Autodesk Fusion 360 part; units mm, degrees
(part 2 of 2)
sketch "Skizze1" plane through (0, 0, 0) normal (0, 0, 1) x (1, 0, 0)
  line L0 (-200, 300) -> (200, 300)
  line L1 (200, 300) -> (200, -300)
  line L2 (200, -300) -> (-200, -300)
  line L3 (-200, -300) -> (-200, 300)
  line L4 (-200, 300) -> (200, -300) construction
  line L5 (200, 300) -> (-200, -300) construction
  dimension "d1" = 600
  dimension "d2" = 400
  constraint horizontal L0
  constraint perpendicular L0 L1
  constraint parallel L0 L2
  constraint parallel L1 L3
  constraint coincident L4 origin
  constraint coincident L5 origin
  measures "d1" distance of L0.end L1.end
  measures "d2" distance of L0.start L0.end
extrude "Extrusion1" add sketch "Skizze1" along normal blind 200
fillet "Abrundung1" radius 40 4 edges at (200, -300, 100) (-200, -300, 100) (200, 300, 100) (-200, 300, 100)
fillet "Abrundung2" radius 5 2 faces at (-66.6667, -86.6667, 200) (-66.6667, -86.6667, 0)
sketch "Skizze2" plane through (0, 0, 200) normal (0, 0, 1) x (-1, 0, 0)
  arc A0 (160, -295) -> (195, -260) centre (160, -260) ccw
  line L0 (195, -260) -> (195, 260)
  arc A1 (195, 260) -> (160, 295) centre (160, 260) ccw
  line L1 (160, 295) -> (-160, 295)
  arc A2 (-160, 295) -> (-195, 260) centre (-160, 260) ccw
  line L2 (-195, 260) -> (-195, -260)
  arc A3 (-195, -260) -> (-160, -295) centre (-160, -260) ccw
  line L3 (-160, -295) -> (160, -295)
  line L4 (-125, -200) -> (125, -200)
  line L5 (125, -200) -> (125, 200)
  line L6 (125, 200) -> (-125, 200)
  line L7 (-125, 200) -> (-125, -200)
  line L8 (-125, -200) -> (125, 200) construction
  line L9 (125, -200) -> (-125, 200) construction
  dimension "d9" = 250
  dimension "d10" = 400
  constraint horizontal L4
  constraint perpendicular L4 L5
  constraint parallel L4 L6
  constraint parallel L5 L7
  constraint coincident L8 origin
  constraint coincident L9 origin
  measures "d9" distance of L4.start L4.end
  measures "d10" distance of L4.start L6.end
hole "Bohrung1" at (125, 200, 200) at (125, -200, 200) direction (0, 0, -1) diameter 30 depth 5 tip angle 180

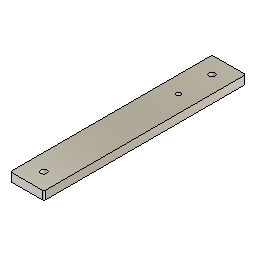
design "StrebeLängs1Cell"
Autodesk Fusion 360 part; units mm, degrees
sketch "Skizze1" plane through (0, 0, 0) normal (0, 0, 1) x (1, 0, 0)
  line L0 (-20, 120) -> (20, 120)
  line L1 (20, 120) -> (20, -120)
  line L2 (20, -120) -> (-20, -120)
  line L3 (-20, -120) -> (-20, 120)
  line L4 (-20, 120) -> (20, -120) construction
  line L5 (20, 120) -> (-20, -120) construction
  dimension "d1" = 40
  dimension "d2" = 240
  constraint horizontal L0
  constraint perpendicular L0 L1
  constraint parallel L0 L2
  constraint parallel L1 L3
  constraint coincident L4 origin
  constraint coincident L5 origin
  measures "d1" distance of L1.end L2.end
  measures "d2" distance of L0.end L1.end
extrude "Extrusion1" add sketch "Skizze1" along normal blind 10
sketch "Skizze2" plane through (0, 0, 10) normal (0, 0, 1) x (-1, 0, 0)
  line L0 (20, 120) -> (-20, 120)
  line L1 (-20, 120) -> (-20, -120)
  line L2 (-20, -120) -> (20, -120)
  line L3 (20, -120) -> (20, 120)
  line L4 (0, -100) -> (0, 100)
  dimension "d5" = 20
  dimension "d6" = 20
  constraint perpendicular L0 L4
  constraint coincident origin L4
  measures "d5" distance of L0 L4.end
  measures "d6" distance of L2 L4.start
hole "Bohrung1" at (0, 100, 10) at (0, -100, 10) direction (0, 0, -1) diameter 7 depth 60 tip angle 118
fillet "Abrundung1" radius 2 4 edges at (-20, -120, 5) (20, -120, 5) (20, 120, 5) (-20, 120, 5)
sketch "Skizze3" plane through (0, 0, 10) normal (0, 0, 1) x (-1, 0, 0)
  circle A0 centre (0, -100) radius 3.5
  circle A1 centre (0, 100) radius 3.5
  arc A2 (18, -120) -> (20, -118) centre (18, -118) ccw
  line L0 (20, -118) -> (20, 118)
  arc A3 (20, 118) -> (18, 120) centre (18, 118) ccw
  line L1 (18, 120) -> (-18, 120)
  arc A4 (-18, 120) -> (-20, 118) centre (-18, 118) ccw
  line L2 (-20, 118) -> (-20, -118)
  arc A5 (-20, -118) -> (-18, -120) centre (-18, -118) ccw
  line L3 (-18, -120) -> (18, -120)
  circle A6 centre (0, -60) radius 9.1766
  dimension "d13" = 60
  measures "d13" distance of origin A6.centre
hole "Bohrung2" at (0, 60, 10) direction (0, 0, -1) diameter 5.035 depth 10 tip angle 118
thread "Gewinde1" "ISO Metric profile 6.0 M6x1 6H"

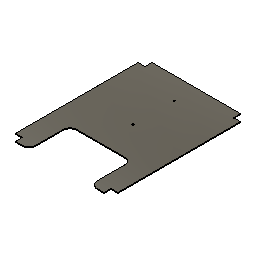
design "MittelPlatte"
Autodesk Fusion 360 part; units mm, degrees
sketch "Skizze1" plane through (0, 0, 0) normal (0, 0, 1) x (1, 0, 0)
  line L0 (-300, 400) -> (300, 400)
  line L1 (300, 400) -> (300, -400)
  line L2 (300, -400) -> (-300, -400)
  line L3 (-300, -400) -> (-300, 400)
  line L4 (-300, 400) -> (300, -400) construction
  line L5 (300, 400) -> (-300, -400) construction
  line L6 (-259.5, 359.5) -> (259.5, 359.5)
  line L7 (259.5, 359.5) -> (259.5, -359.5)
  line L8 (259.5, -359.5) -> (-259.5, -359.5)
  line L9 (-259.5, -359.5) -> (-259.5, 359.5)
  line L10 (-259.5, 359.5) -> (259.5, -359.5) construction
  line L11 (259.5, 359.5) -> (-259.5, -359.5) construction
  line L12 (-300, 400) -> (-259.5, 400)
  line L13 (-259.5, 400) -> (-259.5, 359.5)
  line L14 (-259.5, 359.5) -> (-300, 359.5)
  line L15 (-300, 359.5) -> (-300, 400)
  line L16 (259.5, 359.5) -> (300, 359.5)
  line L17 (300, 359.5) -> (300, 400)
  line L18 (300, 400) -> (259.5, 400)
  line L19 (259.5, 400) -> (259.5, 359.5)
  line L20 (-259.5, -359.5) -> (-300, -359.5)
  line L21 (-300, -359.5) -> (-300, -400)
  line L22 (-300, -400) -> (-259.5, -400)
  line L23 (-259.5, -400) -> (-259.5, -359.5)
  line L24 (259.5, -359.5) -> (300, -359.5)
  line L25 (300, -359.5) -> (300, -400)
  line L26 (300, -400) -> (259.5, -400)
  line L27 (259.5, -400) -> (259.5, -359.5)
  dimension "d1" = 600
  dimension "d2" = 800
  dimension "d3" = 40.5
  dimension "d4" = 40.5
  constraint horizontal L0
  constraint perpendicular L0 L1
  constraint parallel L0 L2
  constraint parallel L1 L3
  constraint coincident L4 origin
  constraint coincident L5 origin
  constraint horizontal L6
  constraint perpendicular L6 L7
  constraint parallel L6 L8
  constraint parallel L7 L9
  constraint coincident L10 origin
  constraint coincident L11 origin
  constraint horizontal L12
  constraint vertical L13
  constraint horizontal L14
  constraint vertical L15
  constraint horizontal L16
  constraint vertical L17
  constraint horizontal L18
  constraint vertical L19
  constraint horizontal L20
  constraint vertical L21
  constraint horizontal L22
  constraint vertical L23
  constraint horizontal L24
  constraint vertical L25
  constraint horizontal L26
  constraint vertical L27
  constraint coincident L0.end L17
  constraint coincident L0 L1.start
  measures "d1" distance of L1.end L2.end
  measures "d2" distance of L0.end L1.end
  measures "d3" distance of L0 L6
  measures "d4" distance of L3 L9
extrude "Extrusion1" add sketch "Skizze1" along normal blind 5 contours L0 L6 L13 L19 | L3 L9 L14 L20 | L6 L7 L8 L9 | L1 L7 L16 L24 | L2 L8 L23 L27
sketch "Skizze4" plane through (0, 0, 5) normal (0, 0, 1) x (-1, 0, 0)
  line L0 (259.5, 400) -> (-259.5, 400)
  line L1 (-259.5, 400) -> (-259.5, 359.5)
  line L2 (-259.5, 359.5) -> (-300, 359.5)
  line L3 (-300, 359.5) -> (-300, -359.5)
  line L4 (-300, -359.5) -> (-259.5, -359.5)
  line L5 (-259.5, -359.5) -> (-259.5, -400)
  line L6 (-259.5, -400) -> (259.5, -400)
  line L7 (259.5, -400) -> (259.5, -359.5)
  line L8 (259.5, -359.5) -> (300, -359.5)
  line L9 (300, -359.5) -> (300, 359.5)
  line L10 (300, 359.5) -> (259.5, 359.5)
  line L11 (259.5, 359.5) -> (259.5, 400)
  line L12 (0, -270) -> (0, -30)
  dimension "d23" = 240
  dimension "d24" = 130
  constraint vertical L12
  constraint coincident origin L12
  measures "d23" distance of L12.start L12.end
  measures "d24" distance of L6 L12.start
hole "Bohrung3" at (0, 270, 5) at (0, 30, 5) direction (0, 0, -1) diameter 10 depth 10 tip angle 118
sketch "Skizze6" plane through (0, 0, 5) normal (0, 0, 1) x (-1, 0, 0)
  line L0 (259.5, -400) -> (259.5, -359.5)
  line L1 (259.5, -359.5) -> (300, -359.5)
  line L2 (300, -359.5) -> (300, 359.5)
  line L3 (300, 359.5) -> (259.5, 359.5)
  line L4 (259.5, 359.5) -> (259.5, 400)
  line L5 (259.5, 400) -> (-259.5, 400)
  line L6 (-259.5, 400) -> (-259.5, 359.5)
  line L7 (-259.5, 359.5) -> (-300, 359.5)
  line L8 (-300, 359.5) -> (-300, -359.5)
  line L9 (-300, -359.5) -> (-259.5, -359.5)
  line L10 (-259.5, -359.5) -> (-259.5, -400)
  line L11 (-259.5, -400) -> (259.5, -400)
  circle A0 centre (0, -270) radius 5
  circle A1 centre (0, -30) radius 5
  line L12 (180, 400) -> (-180, 400)
  line L13 (-180, 400) -> (-180, 160)
  line L14 (-180, 160) -> (180, 160)
  line L15 (180, 160) -> (180, 400)
  line L16 (259.75, 160.25) -> (300.25, 160.25)
  line L17 (300.25, 160.25) -> (300.25, 119.75)
  line L18 (300.25, 119.75) -> (259.75, 119.75)
  line L19 (259.75, 119.75) -> (259.75, 160.25)
  line L20 (259.75, 160.25) -> (300.25, 119.75) construction
  line L21 (300.25, 160.25) -> (259.75, 119.75) construction
  line L22 (-300.25, 160.25) -> (-259.75, 160.25)
  line L23 (-259.75, 160.25) -> (-259.75, 119.75)
  line L24 (-259.75, 119.75) -> (-300.25, 119.75)
  line L25 (-300.25, 119.75) -> (-300.25, 160.25)
  line L26 (-300.25, 160.25) -> (-259.75, 119.75) construction
  line L27 (-259.75, 160.25) -> (-300.25, 119.75) construction
  point P0 (280, 140)
  point P1 (-280, 140)
  dimension "d30" = 560
  dimension "d31" = 120
  dimension "d32" = 120
  dimension "d37" = 40.5
  dimension "d38" = 40.5
  dimension "d39" = 20
  dimension "d40" = 20
  dimension "d42" = 20
  dimension "d43" = 20
  constraint horizontal L12
  constraint vertical L13
  constraint horizontal L14
  constraint vertical L15
  constraint coincident L5 L12.start
  constraint horizontal L16
  constraint perpendicular L16 L17
  constraint parallel L16 L18
  constraint parallel L17 L19
  constraint coincident L20 P0
  constraint coincident L21 P0
  constraint horizontal L22
  constraint perpendicular L22 L23
  constraint parallel L22 L24
  constraint parallel L23 L25
  constraint coincident L26 P1
  constraint coincident L27 P1
  constraint equal L18 L24
  constraint equal L19 L23
  measures "d30" distance of L11 L14
  measures "d31" distance of L2 L15
  measures "d32" distance of L8 L13
  measures "d37" distance of L17.end L18.end
  measures "d38" distance of L16.end L17.end
  measures "d39" distance of L2 P0
  measures "d40" distance of L8 P1
  measures "d42" distance of L14 P1
  measures "d43" distance of L14 P0
extrude "Extrusion2" cut sketch "Skizze6" against normal blind 10 contours L2 L16 L17 L18 | L8 L22 L24 L25 | L5 L12 L13 L14 L15
fillet "Abrundung2" radius 40 4 edges at (-180, -160, 2.5) (180, -160, 2.5) (-180, -400, 2.5) (180, -400, 2.5)
fillet "Abrundung1" radius 2 12 edges at (-300, -359.5, 2.5) (-259.5, -359.5, 2.5) (-259.5, -400, 2.5) (259.5, -400, 2.5) (259.5, -359.5, 2.5) (300, -359.5, 2.5) (300, 359.5, 2.5) (259.5, 359.5, 2.5) (259.5, 400, 2.5) (-300, 359.5, 2.5) (-259.5, 359.5, 2.5) (-259.5, 400, 2.5)
sketch "Skizze5" plane through (0, 0, 5) normal (0, 0, 1) x (-1, 0, 0)
  arc A0 (257.5, -400) -> (259.5, -398) centre (257.5, -398) ccw
  line L0 (259.5, -398) -> (259.5, -361.5)
  arc A1 (261.5, -359.5) -> (259.5, -361.5) centre (261.5, -361.5) ccw
  line L1 (261.5, -359.5) -> (298, -359.5)
  arc A2 (298, -359.5) -> (300, -357.5) centre (298, -357.5) ccw
  line L2 (300, -357.5) -> (300, 357.5)
  arc A3 (300, 357.5) -> (298, 359.5) centre (298, 357.5) ccw
  line L3 (298, 359.5) -> (261.5, 359.5)
  arc A4 (259.5, 361.5) -> (261.5, 359.5) centre (261.5, 361.5) ccw
  line L4 (259.5, 361.5) -> (259.5, 398)
  arc A5 (259.5, 398) -> (257.5, 400) centre (257.5, 398) ccw
  line L5 (-222, 400) -> (-257.5, 400)
  arc A6 (-257.5, 400) -> (-259.5, 398) centre (-257.5, 398) ccw
  line L6 (-259.5, 398) -> (-259.5, 361.5)
  arc A7 (-261.5, 359.5) -> (-259.5, 361.5) centre (-261.5, 361.5) ccw
  line L7 (-261.5, 359.5) -> (-298, 359.5)
  arc A8 (-298, 359.5) -> (-300, 357.5) centre (-298, 357.5) ccw
  line L8 (-300, 357.5) -> (-300, -357.5)
  arc A9 (-300, -357.5) -> (-298, -359.5) centre (-298, -357.5) ccw
  line L9 (-298, -359.5) -> (-261.5, -359.5)
  arc A10 (-259.5, -361.5) -> (-261.5, -359.5) centre (-261.5, -361.5) ccw
  line L10 (-259.5, -361.5) -> (-259.5, -398)
  arc A11 (-259.5, -398) -> (-257.5, -400) centre (-257.5, -398) ccw
  line L11 (-257.5, -400) -> (257.5, -400)
  circle A12 centre (0, -270) radius 5
  circle A13 centre (0, -30) radius 5
  arc A14 (-220, 398) -> (-222, 400) centre (-222, 398) ccw
  line L12 (257.5, 400) -> (222, 400)
  arc A15 (222, 400) -> (220, 398) centre (222, 398) ccw
  line L13 (220, 398) -> (220, 240)
  arc A16 (180, 200) -> (220, 240) centre (180, 240) ccw
  line L14 (180, 200) -> (-180, 200)
  arc A17 (-220, 240) -> (-180, 200) centre (-180, 240) ccw
  line L15 (-220, 240) -> (-220, 398)

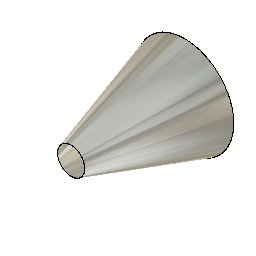
design "Trichter_groß"
Autodesk Fusion 360 part; units mm, degrees
sketch "Skizze1" plane through (0, 0, 0) normal (1, 0, 0) x (0, 1, 0)
  line L0 (-580, 70) -> (-580, 0)
  line L1 (-580, 0) -> (0, 0)
  line L2 (0, 250) -> (0, 0)
  line L3 (-580, 70) -> (0, 250)
  line L4 (-230, 0) -> (-230, 178.6207)
  dimension "d3" = 250
  dimension "d4" = 70
  dimension "d5" = 580
  dimension "d8" = 230
  constraint vertical L0
  constraint perpendicular L0 L1
  constraint perpendicular L1 L2
  constraint coincident L1.end L2
  constraint coincident L2.end L1
  constraint coincident L1 L4.start
  constraint coincident L3 L4.end
  constraint perpendicular L1 L4
  measures "d3" distance of L1.end L2.start
  measures "d4" vertical distance of L1.end L0.start
  measures "d5" distance of L1.end L0
  measures "d8" distance of L2 L4
revolve "Drehen1" add sketch "Skizze1" angle 360 about axis through (0, -580, 0) along (0, 1, 0)
shell "Schale1" thickness 1 removed faces 2 at (33.8089, -580, -13.7168) at (54.8247, 0, 36.3167)

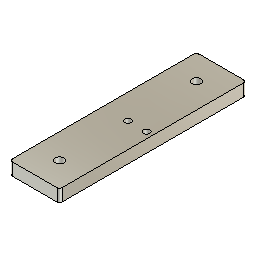
design "StrebeQuer1Cell"
Autodesk Fusion 360 part; units mm, degrees
sketch "Skizze1" plane through (0, 0, 0) normal (0, 0, 1) x (1, 0, 0)
  line L0 (-20, 75) -> (20, 75)
  line L1 (20, 75) -> (20, -75)
  line L2 (20, -75) -> (-20, -75)
  line L3 (-20, -75) -> (-20, 75)
  line L4 (-20, 75) -> (20, -75) construction
  line L5 (20, 75) -> (-20, -75) construction
  dimension "d1" = 40
  dimension "d2" = 150
  constraint horizontal L0
  constraint perpendicular L0 L1
  constraint parallel L0 L2
  constraint parallel L1 L3
  constraint coincident L4 origin
  constraint coincident L5 origin
  measures "d1" distance of L1.end L2.end
  measures "d2" distance of L0.end L1.end
extrude "Extrusion1" add sketch "Skizze1" along normal blind 10
sketch "Skizze2" plane through (0, 0, 10) normal (0, 0, 1) x (-1, 0, 0)
  line L0 (20, 75) -> (-20, 75)
  line L1 (-20, 75) -> (-20, -75)
  line L2 (-20, -75) -> (20, -75)
  line L3 (20, -75) -> (20, 75)
  line L4 (0, -55) -> (0, 55)
  dimension "d5" = 20
  dimension "d6" = 20
  constraint perpendicular L0 L4
  constraint coincident origin L4
  measures "d5" distance of L0 L4.end
  measures "d6" distance of L2 L4.start
hole "Bohrung1" at (0, 55, 10) at (0, -55, 10) direction (0, 0, -1) diameter 7 depth 60 tip angle 118
fillet "Abrundung1" radius 2 4 edges at (-20, -75, 5) (20, -75, 5) (20, 75, 5) (-20, 75, 5)
sketch "Skizze3" plane through (0, 0, 10) normal (0, 0, 1) x (-1, 0, 0)
  circle A0 centre (0, -55) radius 3.5
  circle A1 centre (0, 55) radius 3.5
  arc A2 (18, -75) -> (20, -73) centre (18, -73) ccw
  line L0 (20, -73) -> (20, 73)
  arc A3 (20, 73) -> (18, 75) centre (18, 73) ccw
  line L1 (18, 75) -> (-18, 75)
  arc A4 (-18, 75) -> (-20, 73) centre (-18, 73) ccw
  line L2 (-20, 73) -> (-20, -73)
  arc A5 (-20, -73) -> (-18, -75) centre (-18, -73) ccw
  line L3 (-18, -75) -> (18, -75)
  line L4 (-15, 0) -> (0, 0)
  dimension "d12" = 15
  dimension "d13" = 15
  constraint horizontal L4
  constraint coincident origin L4
  measures "d12" distance of L4.start L4.end
  measures "d13" distance of L4.end L4.start
hole "Bohrung2" at (15, 0, 10) at (0, 0, 10) direction (0, 0, -1) diameter 5 depth 10 tip angle 118

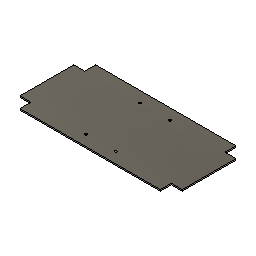
design "WaagePlatte"
Autodesk Fusion 360 part; units mm, degrees
sketch "Skizze1" plane through (0, 0, 0) normal (0, 0, 1) x (1, 0, 0)
  line L0 (-300, 140) -> (300, 140)
  line L1 (300, 140) -> (300, -140)
  line L2 (300, -140) -> (-300, -140)
  line L3 (-300, -140) -> (-300, 140)
  line L4 (-300, 140) -> (300, -140) construction
  line L5 (300, 140) -> (-300, -140) construction
  dimension "d1" = 600
  dimension "d2" = 280
  constraint horizontal L0
  constraint perpendicular L0 L1
  constraint parallel L0 L2
  constraint parallel L1 L3
  constraint coincident L4 origin
  constraint coincident L5 origin
  measures "d1" distance of L1.end L2.end
  measures "d2" distance of L0.end L1.end
extrude "Extrusion1" add sketch "Skizze1" along normal blind 5
sketch "Skizze2" plane through (0, 0, 5) normal (0, 0, 1) x (-1, 0, 0)
  line L0 (300, 140) -> (-300, 140)
  line L1 (-300, 140) -> (-300, -140)
  line L2 (-300, -140) -> (300, -140)
  line L3 (300, -140) -> (300, 140)
  line L4 (259.5, -99.5) -> (-259.5, -99.5)
  line L5 (-259.5, -99.5) -> (-259.5, 99.5)
  line L6 (-259.5, 99.5) -> (259.5, 99.5)
  line L7 (259.5, 99.5) -> (259.5, -99.5)
  line L8 (259.5, -99.5) -> (-259.5, 99.5) construction
  line L9 (-259.5, -99.5) -> (259.5, 99.5) construction
  line L10 (300, -140) -> (259.5, -140)
  line L11 (259.5, -140) -> (259.5, -99.5)
  line L12 (259.5, -99.5) -> (300, -99.5)
  line L13 (300, -99.5) -> (300, -140)
  line L14 (300, 140) -> (259.5, 140)
  line L15 (259.5, 140) -> (259.5, 99.5)
  line L16 (259.5, 99.5) -> (300, 99.5)
  line L17 (300, 99.5) -> (300, 140)
  line L18 (-300, 140) -> (-259.5, 140)
  line L19 (-259.5, 140) -> (-259.5, 99.5)
  line L20 (-259.5, 99.5) -> (-300, 99.5)
  line L21 (-300, 99.5) -> (-300, 140)
  line L22 (-300, -140) -> (-259.5, -140)
  line L23 (-259.5, -140) -> (-259.5, -99.5)
  line L24 (-259.5, -99.5) -> (-300, -99.5)
  line L25 (-300, -99.5) -> (-300, -140)
  dimension "d5" = 40.5
  dimension "d6" = 40.5
  constraint horizontal L4
  constraint perpendicular L4 L5
  constraint parallel L4 L6
  constraint parallel L5 L7
  constraint coincident L8 origin
  constraint coincident L9 origin
  constraint horizontal L10
  constraint vertical L11
  constraint horizontal L12
  constraint vertical L13
  constraint coincident L2.end L3.start
  constraint horizontal L14
  constraint vertical L15
  constraint horizontal L16
  constraint vertical L17
  constraint coincident L0.start L3.end
  constraint horizontal L18
  constraint vertical L19
  constraint horizontal L20
  constraint vertical L21
  constraint coincident L0.end L1.start
  constraint horizontal L22
  constraint vertical L23
  constraint horizontal L24
  constraint vertical L25
  constraint coincident L1.end L2.start
  measures "d5" distance of L3 L7
  measures "d6" distance of L2 L4
extrude "Extrusion2" cut sketch "Skizze2" against normal up to surface (5 mm away) contours L0 L3 L14 L15 L16 L17 | L0 L1 L18 L19 L20 L21 | L2 L3 L10 L11 L12 L13 | L1 L2 L22 L23 L24 L25
sketch "Skizze3" plane through (0, 0, 5) normal (0, 0, 1) x (-1, 0, 0)
  line L0 (259.5, 99.5) -> (259.5, 140)
  line L1 (259.5, 140) -> (-259.5, 140)
  line L2 (-259.5, 140) -> (-259.5, 99.5)
  line L3 (-259.5, 99.5) -> (-300, 99.5)
  line L4 (-300, 99.5) -> (-300, -99.5)
  line L5 (-300, -99.5) -> (-259.5, -99.5)
  line L6 (-259.5, -99.5) -> (-259.5, -140)
  line L7 (-259.5, -140) -> (259.5, -140)
  line L8 (259.5, -140) -> (259.5, -99.5)
  line L9 (259.5, -99.5) -> (300, -99.5)
  line L10 (300, -99.5) -> (300, 99.5)
  line L11 (300, 99.5) -> (259.5, 99.5)
  line L12 (55, -100) -> (-55, -100)
  line L13 (-55, -100) -> (-55, 100)
  line L14 (-55, 100) -> (55, 100)
  line L15 (55, 100) -> (55, -100)
  line L16 (55, -100) -> (-55, 100) construction
  line L17 (-55, -100) -> (55, 100) construction
  dimension "d9" = 110
  dimension "d10" = 200
  constraint horizontal L12
  constraint perpendicular L12 L13
  constraint parallel L12 L14
  constraint parallel L13 L15
  constraint coincident L16 origin
  constraint coincident L17 origin
  measures "d9" distance of L13.end L14.end
  measures "d10" distance of L12.end L13.end
hole "Bohrung1" at (-55, 100, 5) at (55, 100, 5) at (-55, -100, 5) at (55, -100, 5) direction (0, 0, -1) diameter 8.5 depth 100 tip angle 118
fillet "Abrundung1" radius 1 12 edges at (-300, -99.5, 2.5) (-259.5, -99.5, 2.5) (-259.5, -140, 2.5) (259.5, -99.5, 2.5) (300, -99.5, 2.5) (259.5, -140, 2.5) (259.5, 140, 2.5) (259.5, 99.5, 2.5) (300, 99.5, 2.5) (-259.5, 140, 2.5) (-259.5, 99.5, 2.5) (-300, 99.5, 2.5)

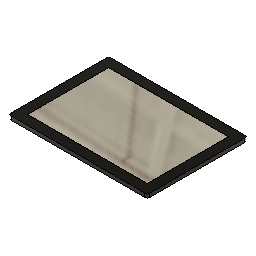
design "Tablet_Lenovo_X1"
Autodesk Fusion 360 part; units mm, degrees
sketch "Skizze1" plane through (0, 0, 0) normal (0, 0, 1) x (1, 0, 0)
  line L0 (-145.5, 105) -> (145.5, 105)
  line L1 (145.5, 105) -> (145.5, -105)
  line L2 (145.5, -105) -> (-145.5, -105)
  line L3 (-145.5, -105) -> (-145.5, 105)
  line L4 (-145.5, 105) -> (145.5, -105) construction
  line L5 (145.5, 105) -> (-145.5, -105) construction
  dimension "d1" = 291
  dimension "d2" = 210
  constraint horizontal L0
  constraint perpendicular L0 L1
  constraint parallel L0 L2
  constraint parallel L1 L3
  constraint coincident L4 origin
  constraint coincident L5 origin
  measures "d1" distance of L1.end L2.end
  measures "d2" distance of L0.end L1.end
extrude "Extrusion1" add sketch "Skizze1" along normal blind 8.9
chamfer "Fase1" distance 1 distance2 8.9 1 faces at (-48.5, -35, 0)
fillet "Abrundung1" radius 5 4 edges at (145, -104.5, 4.45) (145, 104.5, 4.45) (-145, -104.5, 4.45) (-145, 104.5, 4.45)
sketch "Skizze2" plane through (0, 0, 8.9) normal (0, 0, 1) x (-1, 0, 0)
  ellipse E0 centre (140.4685, -99.9685) end of major axis (144.0484, -103.5484) minor radius 5 (140.5313, -105) -> (145.5, -100.0313) ccw
  line L0 (145.5, -100.0313) -> (145.5, 100.0313)
  ellipse E1 centre (140.4685, 99.9685) end of major axis (144.0484, 103.5484) minor radius 5 (145.5, 100.0313) -> (140.5313, 105) ccw
  line L1 (140.5313, 105) -> (-140.5313, 105)
  ellipse E2 centre (-140.4685, 99.9685) end of major axis (-144.0484, 103.5484) minor radius 5 (-140.5313, 105) -> (-145.5, 100.0313) ccw
  line L2 (-145.5, 100.0313) -> (-145.5, -100.0313)
  ellipse E3 centre (-140.4685, -99.9685) end of major axis (-144.0484, -103.5484) minor radius 5 (-145.5, -100.0313) -> (-140.5313, -105) ccw
  line L3 (-140.5313, -105) -> (140.5313, -105)
  line L4 (125.5, -85) -> (-125.5, -85)
  line L5 (-125.5, -85) -> (-125.5, 85)
  line L6 (-125.5, 85) -> (125.5, 85)
  line L7 (125.5, 85) -> (125.5, -85)
  line L8 (125.5, -85) -> (-125.5, 85) construction
  line L9 (-125.5, -85) -> (125.5, 85) construction
  dimension "d9" = 20
  dimension "d10" = 20
  constraint horizontal L4
  constraint perpendicular L4 L5
  constraint parallel L4 L6
  constraint parallel L5 L7
  constraint coincident L8 origin
  constraint coincident L9 origin
  measures "d9" distance of L0 L7
  measures "d10" distance of L3 L4
extrude "Extrusion2" cut sketch "Skizze2" against normal blind 0.1 contours L4 L5 L6 L7
